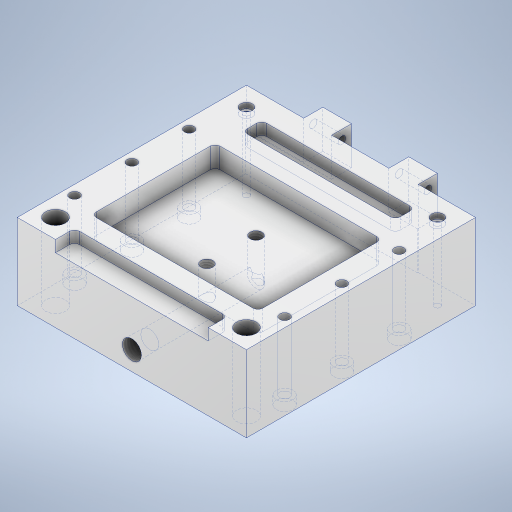
# Autodesk Inventor part: Base - V1
Saved by Autodesk Inventor 2023 (Build 270158000, 158)
## iProperties
Created: 2022-06-13
Part Number: Base - V1
Material: Aluminum 6061
Document SubType Name: Modeling
Designer: Caleb
Density: 2.7 g/cm^3
Appearance: Aluminum - Flat
Mass: 397.038 g
Surface Area: 211.278 cm^2
Volume: 147.051 cm^3
Author: Caleb
Autodesk Inventor part; units mm, degrees
ref_plane "YZ Plane" through (0, 0, 0) normal (1, 0, 0) x (0, 1, 0)
ref_plane "XZ Plane" through (0, 0, 0) normal (0, 1, 0) x (-1, 0, 0)
ref_plane "XY Plane" through (0, 0, 0) normal (0, 0, 1) x (1, 0, 0)
sketch "Sketch1" plane through (0, 0, 0) normal (0, 1, 0) x (-1, 0, 0)
  line L0 (-38.1, -41.275) -> (38.1, -41.275)
  line L1 (38.1, -41.275) -> (38.1, 41.275)
  line L2 (38.1, 41.275) -> (-38.1, 41.275)
  line L3 (-38.1, 41.275) -> (-38.1, -41.275)
  line L4 (-38.1, -41.275) -> (38.1, 41.275) construction
  line L5 (38.1, -41.275) -> (-38.1, 41.275) construction
  point P0 (0, 0)
  dimension "d0" = 76.2
  dimension "d1" = 82.55
  constraints: 12 end point, 2 midpoint, 2 parallel, 1 horizontal, 1 perpendicular
  measures "d0" distance of L2.end L1.end
  measures "d1" distance of L1.end L0.end
extrude "Extrusion1" add sketch "Sketch1" along normal blind 25.4
sketch "Sketch2" plane through (0, 25.4, 0) normal (0, 1, 0) x (1, 0, 0)
  line L0 (9.525, 34.671) -> (9.525, 41.275)
  line L1 (9.525, 41.275) -> (-9.525, 41.275)
  line L2 (-9.525, 41.275) -> (-9.525, 34.671)
  line L3 (-9.525, 34.671) -> (9.525, 34.671)
  line L4 (9.525, 34.671) -> (-9.525, 41.275) construction
  line L5 (9.525, 41.275) -> (-9.525, 34.671) construction
  line L6 (-38.1, 41.275) -> (-38.1, -41.275) projected
  line L7 (-38.1, 41.275) -> (-19.05, 41.275)
  line L8 (-19.05, 41.275) -> (-19.05, 34.925)
  line L9 (-19.05, 34.925) -> (-38.1, 34.925)
  line L10 (-38.1, 34.925) -> (-38.1, 41.275)
  line L11 (38.1, -41.275) -> (38.1, 41.275) projected
  line L12 (38.1, 41.275) -> (19.05, 41.275)
  line L13 (19.05, 41.275) -> (19.05, 34.925)
  line L14 (19.05, 34.925) -> (38.1, 34.925)
  line L15 (38.1, 34.925) -> (38.1, 41.275)
  line L16 (38.1, 41.275) -> (-38.1, 41.275) projected
  point P0 (0, 0)
  point P1 (0, 37.973)
  dimension "d6" = 9.525
  dimension "d7" = 9.525
  dimension "d8" = 6.35
  dimension "d9" = 19.05
  dimension "d58" = 6.604
  constraints: 28 end point, 6 parallel, 3 perpendicular, 2 horizontal, 2 midpoint, 2 point on line, 1 collinear
  measures "d6" distance between parallel lines of L8 L2
  measures "d7" distance between parallel lines of L0 L13
  measures "d8" distance of L9.end L6.start
  measures "d9" distance of L2.end L0.start
  measures "d58" distance of L1.end L2.end
extrude "Extrusion2" cut sketch "Sketch2" against normal through all
sketch "Sketch3" plane through (19.05, 25.4, -34.925) normal (1, 0, 0) x (0, 0, -1)
  line L0 (-0.254, 0) -> (-0.254, -25.4) projected
  line L1 (6.35, -25.4) -> (-0.254, -25.4)
  line L2 (-0.254, -25.4) -> (-0.254, -12.7)
  line L3 (-0.254, -12.7) -> (6.35, -12.7)
  line L4 (6.35, -12.7) -> (6.35, -25.4)
  point P0 (-34.925, -25.4)
  constraints: 8 end point, 2 parallel, 1 horizontal, 1 midpoint, 1 perpendicular
extrude "Extrusion3" cut sketch "Sketch3" against normal through all
sketch "Sketch4" plane through (19.05, 25.4, -34.925) normal (1, 0, 0) x (0, 0, -1)
  line L0 (0, 0) -> (6.35, 0) projected
  line L1 (6.35, 0) -> (6.35, -12.7) projected
  point P0 (-34.925, -25.4)
  point P1 (3.175, -3.175)
  dimension "d14" = 3.175
  dimension "d15" = 3.175
  measures "d14" distance from line of L0 point (3.175, -3.175)
  measures "d15" distance from line of point (3.175, -3.175) L1
hole "Hole1" at (19.05, 22.225, -38.1) direction (-1, 0, 0) diameter 2.54 end through all
sketch "Sketch6" plane through (0, 25.4, 0) normal (0, 1, 0) x (1, 0, 0)
  line L0 (-23.8125, 27.305) -> (23.8125, 27.305)
  line L1 (25.4, 25.7175) -> (25.4, 22.5425)
  line L2 (23.8125, 20.955) -> (-23.8125, 20.955)
  line L3 (-25.4, 22.5425) -> (-25.4, 25.7175)
  line L4 (-38.1, 34.925) -> (-38.1, -41.275) projected
  line L5 (-38.1, -41.275) -> (38.1, -41.275) projected
  line L6 (-25.4, -41.275) -> (25.4, -41.275)
  line L7 (25.4, -41.275) -> (25.4, -36.5125)
  line L8 (23.8125, -34.925) -> (-23.8125, -34.925)
  line L9 (-25.4, -36.5125) -> (-25.4, -41.275)
  arc A0 (-23.8125, -34.925) -> (-25.4, -36.5125) centre (-23.8125, -36.5125) ccw
  arc A1 (25.4, -36.5125) -> (23.8125, -34.925) centre (23.8125, -36.5125) ccw
  arc A2 (23.8125, 20.955) -> (25.4, 22.5425) centre (23.8125, 22.5425) ccw
  arc A3 (25.4, 25.7175) -> (23.8125, 27.305) centre (23.8125, 25.7175) ccw
  arc A4 (-23.8125, 27.305) -> (-25.4, 25.7175) centre (-23.8125, 25.7175) ccw
  arc A5 (-25.4, 22.5425) -> (-23.8125, 20.955) centre (-23.8125, 22.5425) ccw
  line L10 (-19.05, 34.925) -> (-38.1, 34.925) projected
  point P0 (0, 0)
  point P1 (-25.4, 27.305)
  point P2 (-38.1, 31.75)
  point P3 (38.1, 31.75)
  point P4 (25.4, 20.955)
  point P5 (25.4, 27.305)
  point P6 (-25.4, 20.955)
  point P7 (25.4, -34.925)
  point P8 (-25.4, -34.925)
  point P9 (25.4, -41.275)
  dimension "d25" = 50.8
  dimension "d26" = 6.35
  dimension "d28" = 12.7
  dimension "d29" = 50.8
  dimension "d30" = 6.35
  dimension "d31" = 12.7
  dimension "d46" = 1.5875
  dimension "d60" = 7.62
  constraints: 16 end point, 13 point on line, 12 point on circle, 12 tangent, 6 centre point, 5 equal radius, 4 parallel, 2 horizontal, 2 perpendicular
  measures "d25" distance of point (25.4, 20.955) point (-25.4, 20.955)
  measures "d26" distance of point (25.4, 27.305) point (25.4, 20.955)
  measures "d28" distance between parallel lines of L4 L3
  measures "d29" distance of point (-25.4, -34.925) point (25.4, -34.925)
  measures "d30" distance of point (25.4, -34.925) L6.end
  measures "d31" distance between parallel lines of L4 L9
  measures "d46" radius of A0
  measures "d60" distance between parallel lines of L10 L0
extrude "Extrusion5" cut sketch "Sketch6" against normal blind 3.81
sketch "Sketch8" plane through (0, 25.4, 0) normal (0, 1, 0) x (1, 0, 0)
  line L0 (-38.1, 34.925) -> (-38.1, -41.275) projected
  line L1 (-38.1, -41.275) -> (-25.4, -41.275) projected
  line L2 (38.1, -41.275) -> (38.1, 34.925) projected
  line L3 (38.1, 34.925) -> (19.05, 34.925) projected
  point P0 (0, 0)
  point P1 (-31.75, 28.575)
  point P2 (31.75, 28.575)
  dimension "d50" = 6.35
  dimension "d61" = 6.35
  constraints: 1 horizontal alignment
  measures "d50" distance from line of L2 point (31.75, 28.575)
  measures "d61" distance from line of L3 point (31.75, 28.575)
hole "Hole3" at (-31.75, 25.4, -28.575) at (31.75, 25.4, -28.575) direction (0, -1, 0) diameter 2.0574 end through all counterbore diameter 3.9624 counterbore depth 1.8542 clearance for "Socket Head Cap Screw" size "#1" standard "Ansi Unified Screw Threads"
sketch "Sketch9" plane through (0, 25.4, 0) normal (0, 1, 0) x (1, 0, 0)
  line L0 (27.2575, -28.21) -> (-24.9715, -28.21)
  line L1 (-26.559, -26.6225) -> (-26.559, 11.3825)
  line L2 (-24.9715, 12.97) -> (27.2575, 12.97)
  line L3 (28.845, 11.3825) -> (28.845, -26.6225)
  line L4 (38.1, -41.275) -> (38.1, 34.925) projected
  line L5 (25.4, -41.275) -> (38.1, -41.275) projected
  arc A0 (-24.9715, 12.97) -> (-26.559, 11.3825) centre (-24.9715, 11.3825) ccw
  arc A1 (-26.559, -26.6225) -> (-24.9715, -28.21) centre (-24.9715, -26.6225) ccw
  arc A2 (27.2575, -28.21) -> (28.845, -26.6225) centre (27.2575, -26.6225) ccw
  arc A3 (28.845, 11.3825) -> (27.2575, 12.97) centre (27.2575, 11.3825) ccw
  point P0 (0, 0)
  point P1 (28.845, -28.21)
  point P2 (-26.559, 12.97)
  point P3 (-26.559, -28.21)
  point P4 (28.845, 12.97)
  dimension "d62" = 9.255
  dimension "d63" = 13.065
  dimension "d64" = 55.404
  dimension "d65" = 41.18
  dimension "d68" = 1.5875
  constraints: 8 end point, 8 point on circle, 8 point on line, 8 tangent, 4 centre point, 3 equal radius, 2 parallel, 1 horizontal, 1 perpendicular
  measures "d62" distance between parallel lines of L3 L4
  measures "d63" distance between parallel lines of L0 L5
  measures "d64" distance of point (28.845, -28.21) point (-26.559, -28.21)
  measures "d65" distance of point (-26.559, -28.21) point (-26.559, 12.97)
  measures "d68" radius of A0
extrude "Extrusion6" cut sketch "Sketch9" against normal blind 6.8
sketch "Sketch11" plane through (0, 25.4, 0) normal (0, 1, 0) x (1, 0, 0)
  line L0 (-38.1, -41.275) -> (-25.4, -41.275) projected
  line L1 (-38.1, 34.925) -> (-38.1, -41.275) projected
  line L2 (38.1, -41.275) -> (38.1, 34.925) projected
  point P0 (0, 0)
  point P1 (-31.75, -34.925)
  point P2 (31.75, -34.925)
  dimension "d69" = 6.35
  dimension "d70" = 6.35
  dimension "d71" = 6.35
  constraints: 1 horizontal alignment
  measures "d69" distance from line of L0 point (-31.75, -34.925)
  measures "d70" distance from line of L1 point (-31.75, -34.925)
  measures "d71" distance from line of L2 point (31.75, -34.925)
hole "Hole4" at (-31.75, 25.4, 34.925) at (31.75, 25.4, 34.925) direction (0, -1, 0) diameter 6.604 end through all
sketch "Sketch12" plane through (0, 0, 0) normal (0, -1, 0) x (1, 0, 0)
  line L0 (-38.1, -34.671) -> (-38.1, 41.275) projected
  line L1 (-38.1, 41.275) -> (38.1, 41.275) projected
  line L2 (0, 41.275) -> (0, -34.671)
  line L3 (9.525, -34.671) -> (-9.525, -34.671) projected
  point P0 (0, 0)
  point P1 (-34.925, 25.4)
  point P2 (-34.925, 6.35)
  point P3 (-34.925, -12.7)
  point P4 (34.925, 25.4)
  point P5 (34.925, 6.35)
  point P6 (34.925, -12.7)
  dimension "d79" = 3.175
  dimension "d80" = 34.925
  dimension "d81" = 19.05
  dimension "d82" = 19.05
  constraints: 3 symmetric about line, 2 end point, 2 midpoint, 2 vertical alignment
  measures "d79" distance from line of L0 point (-34.925, -12.7)
  measures "d80" distance from line of L1 point (-34.925, 6.35)
  measures "d81" distance of point (-34.925, 25.4) point (-34.925, 6.35)
  measures "d82" distance of point (-34.925, -12.7) point (-34.925, 6.35)
hole "Hole5" at (-34.925, 0, 25.4) at (-34.925, 0, 6.35) at (-34.925, 0, -12.7) at (34.925, 0, -12.7) at (34.925, 0, 6.35) at (34.925, 0, 25.4) direction (0, 1, 0) diameter 3.2766 end through all counterbore diameter 5.5626 counterbore depth 2.8448 clearance for "Socket Head Cap Screw" size "#4" standard "Ansi Unified Screw Threads"
sketch "Sketch13" plane through (0, 18.6, 0) normal (0, 1, 0) x (1, 0, 0)
  point P0 (0, 0)
  point P1 (0, -16.317)
  point P2 (0, 0)
  constraints: 1 coincident, 1 vertical alignment
hole "Hole6" at (0, 18.6, 16.317) at (0, 18.6, 0) direction (0, -1, 0) diameter 3.9624 depth 13.6144 tip angle 118 thread size "10-32 UNF" class "2B" standard "ANSI Unified Screw Threads"
sketch "Sketch14" plane through (-38.1, 0, 41.275) normal (0, 0, 1) x (1, 0, 0)
  line L0 (36.1188, 18.6) -> (40.0812, 18.6) projected
  line L1 (0, 0) -> (76.2, 0) projected
  point P0 (38.1, 0)
  point P1 (38.1, 6.35)
  point P2 (38.1, 0)
  dimension "d97" = 6.35
  constraints: 1 midpoint
  measures "d97" distance of point (38.1, 0) point (38.1, 6.35)
hole "Hole7" at (0, 6.35, 41.275) direction (0, 0, -1) diameter 5.9436 depth 41.275 tip angle 118 taper from width 6.3651 to width 5.9936 over 5.9461 thread size "1/16" designation "1/16 - 27 NPT" standard "NPT for PVC Pipe and Fitting"
equation "\"d7\" = d6"
equation "\"d15\" = d14"
equation "\"d31\" = d28"
equation "\"d50\" = d48"
equation "\"d61\" = d48"
equation "\"d71\" = d70"
equation "\"d82\" = d81"
equation "\"d48\" = 6.35"
body "Solid1"
